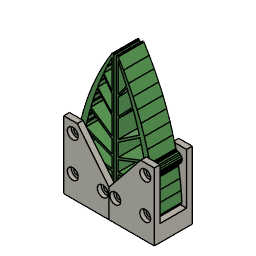
Robotiq_2F85_UMI_Handed (Autodesk Fusion 360 design; units mm, degrees)
part number: 2026-08-28-16-47-17-434
part number: 2026-08-28-16-47-31-177
part number: 2026-08-28-16-47-37-019
Autodesk Fusion 360 part; units mm, degrees
sketch "Single continuous Robotiq-to-UMI adapter envelope" plane through (0, 0, 0) normal (1, 0, 0) x (0, 0, -1) in component "LEFT handed finger"
  line L0 (1.5, 0) -> (-25.7, 0)
  line L1 (-25.7, 0) -> (-25.7, 40.5)
  line L2 (-25.7, 40.5) -> (-17.5, 40.5)
  line L3 (-17.5, 40.5) -> (1.5, 17)
  line L4 (1.5, 17) -> (1.5, 0)
extrude "Extrude1" add sketch "Single continuous Robotiq-to-UMI adapter envelope" along normal mid plane 22.8 makes body 1 in component "LEFT handed finger"
sketch "Continuous TPU pocket - 0.20 mm clearance per side" plane through (0, 0, 0) normal (0, 0, 1) x (1, 0, 0) in component "LEFT handed finger"
  line L0 (-7.94, 10) -> (7.94, 10)
  line L1 (7.94, 10) -> (7.94, 100)
  line L2 (7.94, 100) -> (-7.94, 100)
  line L3 (-7.94, 100) -> (-7.94, 10)
extrude "Extrude2" cut sketch "Continuous TPU pocket - 0.20 mm clearance per side" along normal mid plane 100 bodies 1 in component "LEFT handed finger"
sketch "Exact Robotiq M5 and indexing interface" plane through (0, 0, 0) normal (0, 1, 0) x (1, 0, 0) in component "LEFT handed finger"
  circle A0 centre (0, -12.36) radius 2.65
  circle A1 centre (-4.5, -12.36) radius 1
  circle A2 centre (4.5, -12.36) radius 1
extrude "Extrude3" cut sketch "Exact Robotiq M5 and indexing interface" along normal blind 4 contours A0 bodies 1 in component "LEFT handed finger"
extrude "Extrude4" cut sketch "Exact Robotiq M5 and indexing interface" along normal blind 2.5 contours A1 | A2 bodies 1 in component "LEFT handed finger"
ref_plane "WorkPlane1" through (0, 4, 0) normal (0, 1, 0) x (0, 0, 1) in component "LEFT handed finger"
sketch "Robotiq M5 SHCS head pocket - 9.2 mm" plane through (0, 4, 0) normal (0, 1, 0) x (1, 0, 0) in component "LEFT handed finger"
  circle A0 centre (0, -12.36) radius 4.6
extrude "Extrude5" cut sketch "Robotiq M5 SHCS head pocket - 9.2 mm" along normal blind 6 bodies 1 in component "LEFT handed finger"
sketch "Three UMI M3 holder clearances - 3.6 mm" plane through (0, 0, 0) normal (1, 0, 0) x (0, 0, -1) in component "LEFT handed finger"
  circle A0 centre (-2.25, 13) radius 1.8
  circle A1 centre (-20.25, 13) radius 1.8
  circle A2 centre (-20.25, 34) radius 1.8
extrude "Extrude6" cut sketch "Three UMI M3 holder clearances - 3.6 mm" along normal mid plane 30 bodies 1 in component "LEFT handed finger"
ref_plane "WorkPlane2" through (11.4, 0, 0) normal (1, 0, 0) x (0, 1, 0) in component "LEFT handed finger"
sketch "Three enclosed UMI M3 SHCS head pockets - 6.5 mm" plane through (11.4, 0, 0) normal (1, 0, 0) x (0, 0, -1) in component "LEFT handed finger"
  circle A0 centre (-2.25, 13) radius 3.25
  circle A1 centre (-20.25, 13) radius 3.25
  circle A2 centre (-20.25, 34) radius 3.25
extrude "Extrude7" cut sketch "Three enclosed UMI M3 SHCS head pockets - 6.5 mm" against normal blind 2.4 bodies 1 in component "LEFT handed finger"
ref_plane "WorkPlane3" through (-11.4, 0, 0) normal (1, 0, 0) x (0, 1, 0) in component "LEFT handed finger"
sketch "Three enclosed UMI M3 captive-nut pockets - 6.3 mm AF" plane through (-11.4, 0, 0) normal (1, 0, 0) x (0, 0, -1) in component "LEFT handed finger"
  line L0 (-2.25, 16.6373) -> (-5.4, 14.8187)
  line L1 (-5.4, 14.8187) -> (-5.4, 11.1813)
  line L2 (-5.4, 11.1813) -> (-2.25, 9.3627)
  line L3 (-2.25, 9.3627) -> (0.9, 11.1813)
  line L4 (0.9, 11.1813) -> (0.9, 14.8187)
  line L5 (0.9, 14.8187) -> (-2.25, 16.6373)
  line L6 (-20.25, 16.6373) -> (-23.4, 14.8187)
  line L7 (-23.4, 14.8187) -> (-23.4, 11.1813)
  line L8 (-23.4, 11.1813) -> (-20.25, 9.3627)
  line L9 (-20.25, 9.3627) -> (-17.1, 11.1813)
  line L10 (-17.1, 11.1813) -> (-17.1, 14.8187)
  line L11 (-17.1, 14.8187) -> (-20.25, 16.6373)
  line L12 (-20.25, 37.6373) -> (-23.4, 35.8187)
  line L13 (-23.4, 35.8187) -> (-23.4, 32.1813)
  line L14 (-23.4, 32.1813) -> (-20.25, 30.3627)
  line L15 (-20.25, 30.3627) -> (-17.1, 32.1813)
  line L16 (-17.1, 32.1813) -> (-17.1, 35.8187)
  line L17 (-17.1, 35.8187) -> (-20.25, 37.6373)
extrude "Extrude8" cut sketch "Three enclosed UMI M3 captive-nut pockets - 6.3 mm AF" along normal blind 2.5 bodies 1 in component "LEFT handed finger"
sketch "Exact 0.600 UMI exterior at zero-gap datum" plane through (0, 0, 0) normal (1, 0, 0) x (0, 0, -1) in component "LEFT handed finger"
  line L0 (-21.2844, 10) -> (-0.9715, 10.0017)
  line L1 (-0.9715, 10.0017) -> (-0.4344, 10.1086)
  line L2 (-0.4344, 10.1086) -> (0.0764, 10.3965)
  line L3 (0.0764, 10.3965) -> (0.4681, 10.8329)
  line L4 (0.4681, 10.8329) -> (0.6887, 11.3341)
  line L5 (0.6887, 11.3341) -> (0.75, 11.8)
  line L6 (0.75, 11.8) -> (0.75, 83.4188)
  line L7 (0.75, 83.4188) -> (0.7057, 83.6451)
  line L8 (0.7057, 83.6451) -> (0.5792, 83.838)
  line L9 (0.5792, 83.838) -> (0.3894, 83.969)
  line L10 (0.3894, 83.969) -> (0.1513, 84.0187)
  line L11 (0.1513, 84.0187) -> (-0.1335, 83.9476)
  line L12 (-0.1335, 83.9476) -> (-0.3574, 83.739)
  line L13 (-0.3574, 83.739) -> (-3.5477, 78.4418)
  line L14 (-3.5477, 78.4418) -> (-6.5147, 73.0163)
  line L15 (-6.5147, 73.0163) -> (-9.2532, 67.472)
  line L16 (-9.2532, 67.472) -> (-11.7585, 61.8185)
  line L17 (-11.7585, 61.8185) -> (-14.0262, 56.0656)
  line L18 (-14.0262, 56.0656) -> (-16.0523, 50.2232)
  line L19 (-16.0523, 50.2232) -> (-17.8334, 44.3015)
  line L20 (-17.8334, 44.3015) -> (-19.4939, 37.9469)
  line L21 (-19.4939, 37.9469) -> (-19.7702, 37.5295)
  line L22 (-19.7702, 37.5295) -> (-20.1502, 37.2037)
  line L23 (-20.1502, 37.2037) -> (-20.4955, 37.0321)
  line L24 (-20.4955, 37.0321) -> (-21.5317, 36.7124)
  line L25 (-21.5317, 36.7124) -> (-22.1844, 36.293)
  line L26 (-22.1844, 36.293) -> (-22.7798, 35.6125)
  line L27 (-22.7798, 35.6125) -> (-23.1454, 34.7854)
  line L28 (-23.1454, 34.7854) -> (-23.2373, 34.2756)
  line L29 (-23.2373, 34.2756) -> (-23.2402, 33.7575)
  line L30 (-23.2402, 33.7575) -> (-23.1539, 33.2467)
  line L31 (-23.1539, 33.2467) -> (-22.981, 32.7584)
  line L32 (-22.981, 32.7584) -> (-22.487, 32.001)
  line L33 (-22.487, 32.001) -> (-21.4511, 31.0732)
  line L34 (-21.4511, 31.0732) -> (-21.1951, 30.599)
  line L35 (-21.1951, 30.599) -> (-21.0961, 30.1474)
  line L36 (-21.0961, 30.1474) -> (-21.1039, 29.7619)
  line L37 (-21.1039, 29.7619) -> (-22.0094, 23.7815)
  line L38 (-22.0094, 23.7815) -> (-22.6654, 17.8463)
  line L39 (-22.6654, 17.8463) -> (-23.0844, 11.8128)
  line L40 (-23.0844, 11.8128) -> (-22.9582, 11.1378)
  line L41 (-22.9582, 11.1378) -> (-22.7802, 10.7986)
  line L42 (-22.7802, 10.7986) -> (-22.5344, 10.5048)
  line L43 (-22.5344, 10.5048) -> (-21.9584, 10.131)
  line L44 (-21.9584, 10.131) -> (-21.2844, 10)
extrude "Extrude9" add sketch "Exact 0.600 UMI exterior at zero-gap datum" along normal mid plane 15.48 separate body makes body 2 in component "LEFT handed finger"
sketch "Six unchanged UMI-derived through-bays" plane through (0, 0, 0) normal (1, 0, 0) x (0, 0, -1) in component "LEFT handed finger"
  line L0 (-18.498, 16) -> (-0.33, 16)
  line L1 (-0.33, 16) -> (-0.33, 22.564)
  line L2 (-0.33, 22.564) -> (-18.18, 25.258)
  line L3 (-18.18, 25.258) -> (-18.516, 22.738)
  line L4 (-18.516, 22.738) -> (-18.66, 21.544)
  line L5 (-18.66, 21.544) -> (-18.942, 19)
  line L6 (-18.942, 19) -> (-19.062, 17.8)
  line L7 (-19.062, 17.8) -> (-19.23, 16)
  line L8 (-19.23, 16) -> (-18.498, 16)
  line L9 (-18.012, 26.446) -> (-0.33, 23.782)
  line L10 (-0.33, 23.782) -> (-0.33, 30.214)
  line L11 (-0.33, 30.214) -> (-16.242, 36.46)
  line L12 (-16.242, 36.46) -> (-16.758, 33.88)
  line L13 (-16.758, 33.88) -> (-16.98, 32.692)
  line L14 (-16.98, 32.692) -> (-17.424, 30.154)
  line L15 (-17.424, 30.154) -> (-17.622, 28.966)
  line L16 (-17.622, 28.966) -> (-18.012, 26.446)
  line L17 (-15.99, 37.648) -> (-0.33, 31.504)
  line L18 (-0.33, 31.504) -> (-0.33, 39.364)
  line L19 (-0.33, 39.364) -> (-13.38, 48.256)
  line L20 (-13.38, 48.256) -> (-14.148, 45.424)
  line L21 (-14.148, 45.424) -> (-14.46, 44.218)
  line L22 (-14.46, 44.218) -> (-15.126, 41.488)
  line L23 (-15.126, 41.488) -> (-15.408, 40.288)
  line L24 (-15.408, 40.288) -> (-15.99, 37.648)
  line L25 (-13.032, 49.474) -> (-0.33, 40.816)
  line L26 (-0.33, 40.816) -> (-0.33, 51.628)
  line L27 (-0.33, 51.628) -> (-9.264, 61.084)
  line L28 (-9.264, 61.084) -> (-10.5, 57.562)
  line L29 (-10.5, 57.562) -> (-10.752, 56.818)
  line L30 (-10.752, 56.818) -> (-11.772, 53.68)
  line L31 (-11.772, 53.68) -> (-12.15, 52.45)
  line L32 (-12.15, 52.45) -> (-13.032, 49.474)
  line L33 (-8.982, 61.84) -> (-0.33, 52.678)
  line L34 (-0.33, 52.678) -> (-0.33, 62.842)
  line L35 (-0.33, 62.842) -> (-5.646, 70.222)
  line L36 (-5.646, 70.222) -> (-7.266, 66.31)
  line L37 (-7.266, 66.31) -> (-7.572, 65.548)
  line L38 (-7.572, 65.548) -> (-8.982, 61.84)
  line L39 (-5.316, 70.99) -> (-0.33, 64.078)
  line L40 (-0.33, 64.078) -> (-0.33, 81.52)
  line L41 (-0.33, 81.52) -> (-3.09, 75.91)
  line L42 (-3.09, 75.91) -> (-3.456, 75.13)
  line L43 (-3.456, 75.13) -> (-5.316, 70.99)
extrude "Extrude10" cut sketch "Six unchanged UMI-derived through-bays" along normal mid plane 24 bodies 2 in component "LEFT handed finger"
sketch "Three UMI TPU M3 clearances - 4.0 mm" plane through (0, 0, 0) normal (1, 0, 0) x (0, 0, -1) in component "LEFT handed finger"
  circle A0 centre (-2.25, 13) radius 2
  circle A1 centre (-20.25, 13) radius 2
  circle A2 centre (-20.25, 34) radius 2
extrude "Extrude11" cut sketch "Three UMI TPU M3 clearances - 4.0 mm" along normal mid plane 24 bodies 2 in component "LEFT handed finger"
sketch "Single continuous Robotiq-to-UMI adapter envelope (2)" plane through (0, 0, 0) normal (1, 0, 0) x (0, 0, -1) in component "RIGHT handed finger"
  line L0 (1.5, 0) -> (-25.7, 0)
  line L1 (-25.7, 0) -> (-25.7, 40.5)
  line L2 (-25.7, 40.5) -> (-17.5, 40.5)
  line L3 (-17.5, 40.5) -> (1.5, 17)
  line L4 (1.5, 17) -> (1.5, 0)
extrude "Extrude1'" add sketch "Single continuous Robotiq-to-UMI adapter envelope (2)" along normal mid plane 22.8 separate body makes body 3 in component "RIGHT handed finger"
sketch "Continuous TPU pocket - 0.20 mm clearance per side (2)" plane through (0, 0, 0) normal (0, 0, 1) x (1, 0, 0) in component "RIGHT handed finger"
  line L0 (-7.94, 10) -> (7.94, 10)
  line L1 (7.94, 10) -> (7.94, 100)
  line L2 (7.94, 100) -> (-7.94, 100)
  line L3 (-7.94, 100) -> (-7.94, 10)
extrude "Extrude2'" cut sketch "Continuous TPU pocket - 0.20 mm clearance per side (2)" along normal mid plane 100 bodies 3 in component "RIGHT handed finger"
sketch "Exact Robotiq M5 and indexing interface (2)" plane through (0, 0, 0) normal (0, 1, 0) x (1, 0, 0) in component "RIGHT handed finger"
  circle A0 centre (0, -12.36) radius 2.65
  circle A1 centre (-4.5, -12.36) radius 1
  circle A2 centre (4.5, -12.36) radius 1
extrude "Extrude3'" cut sketch "Exact Robotiq M5 and indexing interface (2)" along normal blind 4 contours A0 bodies 3 in component "RIGHT handed finger"
extrude "Extrude4'" cut sketch "Exact Robotiq M5 and indexing interface (2)" along normal blind 2.5 contours A1 | A2 bodies 3 in component "RIGHT handed finger"
ref_plane "WorkPlane1" through (0, 4, 0) normal (0, 1, 0) x (0, 0, 1) in component "RIGHT handed finger"
sketch "Robotiq M5 SHCS head pocket - 9.2 mm (2)" plane through (0, 4, 0) normal (0, 1, 0) x (1, 0, 0) in component "RIGHT handed finger"
  circle A0 centre (0, -12.36) radius 4.6
extrude "Extrude5'" cut sketch "Robotiq M5 SHCS head pocket - 9.2 mm (2)" along normal blind 6 bodies 3 in component "RIGHT handed finger"
sketch "Three UMI M3 holder clearances - 3.6 mm (2)" plane through (0, 0, 0) normal (1, 0, 0) x (0, 0, -1) in component "RIGHT handed finger"
  circle A0 centre (-2.25, 13) radius 1.8
  circle A1 centre (-20.25, 13) radius 1.8
  circle A2 centre (-20.25, 34) radius 1.8
extrude "Extrude6'" cut sketch "Three UMI M3 holder clearances - 3.6 mm (2)" along normal mid plane 30 bodies 3 in component "RIGHT handed finger"
ref_plane "WorkPlane2" through (-11.4, 0, 0) normal (1, 0, 0) x (0, 1, 0) in component "RIGHT handed finger"
sketch "Three enclosed UMI M3 SHCS head pockets - 6.5 mm (2)" plane through (-11.4, 0, 0) normal (1, 0, 0) x (0, 0, -1) in component "RIGHT handed finger"
  circle A0 centre (-2.25, 13) radius 3.25
  circle A1 centre (-20.25, 13) radius 3.25
  circle A2 centre (-20.25, 34) radius 3.25
extrude "Extrude7'" cut sketch "Three enclosed UMI M3 SHCS head pockets - 6.5 mm (2)" along normal blind 2.4 bodies 3 in component "RIGHT handed finger"
ref_plane "WorkPlane3" through (11.4, 0, 0) normal (1, 0, 0) x (0, 1, 0) in component "RIGHT handed finger"
sketch "Three enclosed UMI M3 captive-nut pockets - 6.3 mm AF (2)" plane through (11.4, 0, 0) normal (1, 0, 0) x (0, 0, -1) in component "RIGHT handed finger"
  line L0 (-2.25, 16.6373) -> (-5.4, 14.8187)
  line L1 (-5.4, 14.8187) -> (-5.4, 11.1813)
  line L2 (-5.4, 11.1813) -> (-2.25, 9.3627)
  line L3 (-2.25, 9.3627) -> (0.9, 11.1813)
  line L4 (0.9, 11.1813) -> (0.9, 14.8187)
  line L5 (0.9, 14.8187) -> (-2.25, 16.6373)
  line L6 (-20.25, 16.6373) -> (-23.4, 14.8187)
  line L7 (-23.4, 14.8187) -> (-23.4, 11.1813)
  line L8 (-23.4, 11.1813) -> (-20.25, 9.3627)
  line L9 (-20.25, 9.3627) -> (-17.1, 11.1813)
  line L10 (-17.1, 11.1813) -> (-17.1, 14.8187)
  line L11 (-17.1, 14.8187) -> (-20.25, 16.6373)
  line L12 (-20.25, 37.6373) -> (-23.4, 35.8187)
  line L13 (-23.4, 35.8187) -> (-23.4, 32.1813)
  line L14 (-23.4, 32.1813) -> (-20.25, 30.3627)
  line L15 (-20.25, 30.3627) -> (-17.1, 32.1813)
  line L16 (-17.1, 32.1813) -> (-17.1, 35.8187)
  line L17 (-17.1, 35.8187) -> (-20.25, 37.6373)
extrude "Extrude8'" cut sketch "Three enclosed UMI M3 captive-nut pockets - 6.3 mm AF (2)" against normal blind 2.5 bodies 3 in component "RIGHT handed finger"
sketch "Exact 0.600 UMI exterior at zero-gap datum (2)" plane through (0, 0, 0) normal (1, 0, 0) x (0, 0, -1) in component "RIGHT handed finger"
  line L0 (-21.2844, 10) -> (-0.9715, 10.0017)
  line L1 (-0.9715, 10.0017) -> (-0.4344, 10.1086)
  line L2 (-0.4344, 10.1086) -> (0.0764, 10.3965)
  line L3 (0.0764, 10.3965) -> (0.4681, 10.8329)
  line L4 (0.4681, 10.8329) -> (0.6887, 11.3341)
  line L5 (0.6887, 11.3341) -> (0.75, 11.8)
  line L6 (0.75, 11.8) -> (0.75, 83.4188)
  line L7 (0.75, 83.4188) -> (0.7057, 83.6451)
  line L8 (0.7057, 83.6451) -> (0.5792, 83.838)
  line L9 (0.5792, 83.838) -> (0.3894, 83.969)
  line L10 (0.3894, 83.969) -> (0.1513, 84.0187)
  line L11 (0.1513, 84.0187) -> (-0.1335, 83.9476)
  line L12 (-0.1335, 83.9476) -> (-0.3574, 83.739)
  line L13 (-0.3574, 83.739) -> (-3.5477, 78.4418)
  line L14 (-3.5477, 78.4418) -> (-6.5147, 73.0163)
  line L15 (-6.5147, 73.0163) -> (-9.2532, 67.472)
  line L16 (-9.2532, 67.472) -> (-11.7585, 61.8185)
  line L17 (-11.7585, 61.8185) -> (-14.0262, 56.0656)
  line L18 (-14.0262, 56.0656) -> (-16.0523, 50.2232)
  line L19 (-16.0523, 50.2232) -> (-17.8334, 44.3015)
  line L20 (-17.8334, 44.3015) -> (-19.4939, 37.9469)
  line L21 (-19.4939, 37.9469) -> (-19.7702, 37.5295)
  line L22 (-19.7702, 37.5295) -> (-20.1502, 37.2037)
  line L23 (-20.1502, 37.2037) -> (-20.4955, 37.0321)
  line L24 (-20.4955, 37.0321) -> (-21.5317, 36.7124)
  line L25 (-21.5317, 36.7124) -> (-22.1844, 36.293)
  line L26 (-22.1844, 36.293) -> (-22.7798, 35.6125)
  line L27 (-22.7798, 35.6125) -> (-23.1454, 34.7854)
  line L28 (-23.1454, 34.7854) -> (-23.2373, 34.2756)
  line L29 (-23.2373, 34.2756) -> (-23.2402, 33.7575)
  line L30 (-23.2402, 33.7575) -> (-23.1539, 33.2467)
  line L31 (-23.1539, 33.2467) -> (-22.981, 32.7584)
  line L32 (-22.981, 32.7584) -> (-22.487, 32.001)
  line L33 (-22.487, 32.001) -> (-21.4511, 31.0732)
  line L34 (-21.4511, 31.0732) -> (-21.1951, 30.599)
  line L35 (-21.1951, 30.599) -> (-21.0961, 30.1474)
  line L36 (-21.0961, 30.1474) -> (-21.1039, 29.7619)
  line L37 (-21.1039, 29.7619) -> (-22.0094, 23.7815)
  line L38 (-22.0094, 23.7815) -> (-22.6654, 17.8463)
  line L39 (-22.6654, 17.8463) -> (-23.0844, 11.8128)
  line L40 (-23.0844, 11.8128) -> (-22.9582, 11.1378)
  line L41 (-22.9582, 11.1378) -> (-22.7802, 10.7986)
  line L42 (-22.7802, 10.7986) -> (-22.5344, 10.5048)
  line L43 (-22.5344, 10.5048) -> (-21.9584, 10.131)
  line L44 (-21.9584, 10.131) -> (-21.2844, 10)
extrude "Extrude9'" add sketch "Exact 0.600 UMI exterior at zero-gap datum (2)" along normal mid plane 15.48 separate body makes body 4 in component "RIGHT handed finger"
sketch "Six unchanged UMI-derived through-bays (2)" plane through (0, 0, 0) normal (1, 0, 0) x (0, 0, -1) in component "RIGHT handed finger"
  line L0 (-18.498, 16) -> (-0.33, 16)
  line L1 (-0.33, 16) -> (-0.33, 22.564)
  line L2 (-0.33, 22.564) -> (-18.18, 25.258)
  line L3 (-18.18, 25.258) -> (-18.516, 22.738)
  line L4 (-18.516, 22.738) -> (-18.66, 21.544)
  line L5 (-18.66, 21.544) -> (-18.942, 19)
  line L6 (-18.942, 19) -> (-19.062, 17.8)
  line L7 (-19.062, 17.8) -> (-19.23, 16)
  line L8 (-19.23, 16) -> (-18.498, 16)
  line L9 (-18.012, 26.446) -> (-0.33, 23.782)
  line L10 (-0.33, 23.782) -> (-0.33, 30.214)
  line L11 (-0.33, 30.214) -> (-16.242, 36.46)
  line L12 (-16.242, 36.46) -> (-16.758, 33.88)
  line L13 (-16.758, 33.88) -> (-16.98, 32.692)
  line L14 (-16.98, 32.692) -> (-17.424, 30.154)
  line L15 (-17.424, 30.154) -> (-17.622, 28.966)
  line L16 (-17.622, 28.966) -> (-18.012, 26.446)
  line L17 (-15.99, 37.648) -> (-0.33, 31.504)
  line L18 (-0.33, 31.504) -> (-0.33, 39.364)
  line L19 (-0.33, 39.364) -> (-13.38, 48.256)
  line L20 (-13.38, 48.256) -> (-14.148, 45.424)
  line L21 (-14.148, 45.424) -> (-14.46, 44.218)
  line L22 (-14.46, 44.218) -> (-15.126, 41.488)
  line L23 (-15.126, 41.488) -> (-15.408, 40.288)
  line L24 (-15.408, 40.288) -> (-15.99, 37.648)
  line L25 (-13.032, 49.474) -> (-0.33, 40.816)
  line L26 (-0.33, 40.816) -> (-0.33, 51.628)
  line L27 (-0.33, 51.628) -> (-9.264, 61.084)
  line L28 (-9.264, 61.084) -> (-10.5, 57.562)
  line L29 (-10.5, 57.562) -> (-10.752, 56.818)
  line L30 (-10.752, 56.818) -> (-11.772, 53.68)
  line L31 (-11.772, 53.68) -> (-12.15, 52.45)
  line L32 (-12.15, 52.45) -> (-13.032, 49.474)
  line L33 (-8.982, 61.84) -> (-0.33, 52.678)
  line L34 (-0.33, 52.678) -> (-0.33, 62.842)
  line L35 (-0.33, 62.842) -> (-5.646, 70.222)
  line L36 (-5.646, 70.222) -> (-7.266, 66.31)
  line L37 (-7.266, 66.31) -> (-7.572, 65.548)
  line L38 (-7.572, 65.548) -> (-8.982, 61.84)
  line L39 (-5.316, 70.99) -> (-0.33, 64.078)
  line L40 (-0.33, 64.078) -> (-0.33, 81.52)
  line L41 (-0.33, 81.52) -> (-3.09, 75.91)
  line L42 (-3.09, 75.91) -> (-3.456, 75.13)
  line L43 (-3.456, 75.13) -> (-5.316, 70.99)
extrude "Extrude10'" cut sketch "Six unchanged UMI-derived through-bays (2)" along normal mid plane 24 bodies 4 in component "RIGHT handed finger"
sketch "Three UMI TPU M3 clearances - 4.0 mm (2)" plane through (0, 0, 0) normal (1, 0, 0) x (0, 0, -1) in component "RIGHT handed finger"
  circle A0 centre (-2.25, 13) radius 2
  circle A1 centre (-20.25, 13) radius 2
  circle A2 centre (-20.25, 34) radius 2
extrude "Extrude11'" cut sketch "Three UMI TPU M3 clearances - 4.0 mm (2)" along normal mid plane 24 bodies 4 in component "RIGHT handed finger"
component "LEFT handed finger" placed x (0, 0, 1) y (0, 1, 0) z (-1, 0, 0) at (-1.5, 124.82, 0)
component "RIGHT handed finger" placed x (0, 0, -1) y (0, 1, 0) z (1, 0, 0) at (1.5, 124.82, 0)
equation "adapterOverallWidth = 22.8 mm" comment "Handed PETG adapter width"
equation "adapterSlotWidth = 15.88 mm" comment "15.48 mm TPU plus 0.20 mm clearance per side"
equation "tpuFingerThickness = 15.48 mm" comment "Exact 0.600 scale of the UMI 25.8 mm thickness"
equation "adapterM3Clearance = 3.6 mm" comment "UMI holder M3 clearance"
equation "tpuM3Clearance = 4.0 mm" comment "UMI soft-finger M3 clearance"
equation "closedClearancePerSide = 0.75 mm" comment "Original accepted 1.5 mm pair gap; grip tape fills it"
equation "m5ShoulderDepth = 4 mm" comment "Unchanged OEM fingertip shoulder"
equation "m5HeadToolPocketDepth = 6 mm" comment "Reduced from 10 mm for the measured 4.9 mm M5 head"
equation "adapterRootDepth = 10 mm" comment "Unchanged 4 mm shoulder plus 6 mm M5 head pocket"
equation "tpuRootShift = -4 mm" comment "Move TPU base from Y=14 mm to the Y=10 mm PETG split"
equation "adapterDistalExtent = 40.5 mm" comment "Trimmed inward from 42.9 mm at the user's marked PETG edge"
equation "d28 = -( 2.4 mm )"
equation "d60 = -( 2.5 mm )"
named bodies: "PETG Adapter LEFT", "TPU 95A Finger LEFT", "PETG Adapter RIGHT", "TPU 95A Finger RIGHT"
